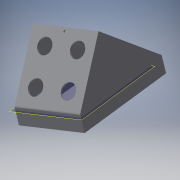
# Autodesk Inventor part: button_angle
Saved by Autodesk Inventor 2016 (Build 200138000, 138)
## iProperties
Created: 2014-10-12
Part Number: button_angle
Material: Generic
Document SubType Name: Modeling
Designer: Alec
Density: 1 g/cm^3
Appearance: Default
Author: Alec
Autodesk Inventor part; units mm, degrees
ref_plane "YZ Plane" through (0, 0, 0) normal (1, 0, 0) x (0, 1, 0)
ref_plane "XZ Plane" through (0, 0, 0) normal (0, 1, 0) x (-1, 0, 0)
ref_plane "XY Plane" through (0, 0, 0) normal (0, 0, 1) x (1, 0, 0)
sketch "Sketch1" plane through (0, 0, 0) normal (0, 1, 0) x (-1, 0, 0)
  line L0 (0, 0) -> (-127, 0)
  line L1 (-127, 0) -> (-127, -6.35)
  line L2 (-127, -6.35) -> (0, -6.35)
  line L3 (0, -6.35) -> (0, 0)
  line L4 (0, -6.35) -> (-6.35, -6.35)
  line L5 (-6.35, -6.35) -> (-6.35, -127)
  line L6 (-6.35, -127) -> (0, -127)
  line L7 (0, -127) -> (0, -6.35)
  line L8 (-127, -6.35) -> (-120.65, -6.35)
  line L9 (-120.65, -6.35) -> (-120.65, -127)
  line L10 (-120.65, -127) -> (-127, -127)
  line L11 (-127, -127) -> (-127, -6.35)
  dimension "d0" = 127
  dimension "d1" = 6.35
  dimension "d2" = 6.35
  dimension "d3" = 120.65
  dimension "d4" = 120.65
  dimension "d5" = 6.35
  constraints: 24 end point, 6 parallel, 3 horizontal, 3 perpendicular
  measures "d0" distance of L1.end L2.end
  measures "d1" distance of L0.end L1.end
  measures "d2" distance of L5.end L6.end
  measures "d3" distance between parallel lines of L2 L6
  measures "d4" distance between parallel lines of L2 L10
  measures "d5" distance between parallel lines of L11 L9
extrude "Extrusion1" add sketch "Sketch1" along normal blind 6.35
sketch "Sketch2" plane through (127, 0, 0) normal (1, 0, 0) x (0, 0, -1)
  line L0 (127, 6.35) -> (120.65, 0)
  line L1 (6.35, 0) -> (127, 0) projected
  line L2 (127, 0) -> (127, 6.35) projected
  line L3 (120.65, 0) -> (127, 0)
  line L4 (127, 0) -> (127, 6.35) projected
  line L5 (127, 6.35) -> (127, 0)
  point P0 (0, 0)
  dimension "d8" = 135
  constraints: 6 end point, 1 collinear, 1 perpendicular, 1 point on line
  measures "d8" angle of L2 L0
extrude "Extrusion2" cut sketch "Sketch2" against normal blind 152.4
sketch "Sketch4" plane through (0, 6.35, 0) normal (0, 1, 0) x (1, 0, 0)
  line L0 (127, 120.65) -> (127, 127)
  line L1 (127, 120.65) -> (127, 127) projected
  line L2 (127, 127) -> (120.65, 127)
  line L3 (120.65, 127) -> (120.65, 120.65)
  line L4 (120.65, 120.65) -> (127, 120.65)
  point P0 (0, 0)
  constraints: 8 end point, 3 perpendicular, 1 collinear
extrude "Extrusion3" cut sketch "Sketch4" against normal blind 152.4
sketch "Sketch5" plane through (0, 6.35, 0) normal (0, 1, 0) x (1, 0, 0)
  line L0 (120.65, 120.65) -> (120.65, 127.0036)
  line L1 (120.65, 127.0036) -> (127.0123, 127.0036)
  line L2 (127.0123, 127.0036) -> (127.0123, 120.65)
  line L3 (127.0123, 120.65) -> (120.65, 120.65)
  point P0 (0, 0)
  constraints: 8 end point, 3 perpendicular, 1 vertical
extrude "Extrusion4" add sketch "Sketch5" against normal blind 152.4
sketch "Sketch6" plane through (0, 6.35, 0) normal (0, 1, 0) x (1, 0, 0)
  line L0 (0, 127) -> (0, 120.65)
  line L1 (0, 127) -> (0, 120.65) projected
  line L2 (0, 120.65) -> (6.35, 120.65)
  line L3 (0, 120.65) -> (6.35, 120.65) projected
  line L4 (6.35, 120.65) -> (6.35, 127)
  line L5 (6.35, 127) -> (0, 127)
  point P0 (0, 0)
  constraints: 8 end point, 2 collinear, 2 perpendicular
extrude "Extrusion5" cut sketch "Sketch6" against normal blind 101.6
sketch "Sketch7" plane through (0, 6.35, 0) normal (0, 1, 0) x (1, 0, 0)
  line L0 (0, 120.65) -> (6.35, 120.65)
  line L1 (6.35, 120.65) -> (6.35, 126.9915)
  line L2 (6.35, 126.9915) -> (0, 126.9915)
  line L3 (0, 126.9915) -> (0, 120.65)
  point P0 (0, 0)
  constraints: 8 end point, 2 parallel, 1 horizontal, 1 perpendicular
extrude "Extrusion6" add sketch "Sketch7" against normal blind 152.4
sketch "Sketch8" plane through (6.35, 0, -6.35) normal (1, 0, 0) x (0, 0, -1)
  line L0 (120.6415, 6.35) -> (120.6415, -146.05) projected
  line L1 (114.3, -146.05) -> (120.6415, -146.05)
  line L2 (120.6415, -146.05) -> (120.6415, -139.7)
  line L3 (120.6415, -139.7) -> (114.3, -139.7)
  line L4 (114.3, -139.7) -> (114.3, -146.05)
  point P0 (-6.35, 0)
  dimension "d19" = 6.35
  constraints: 8 end point, 2 parallel, 1 horizontal, 1 perpendicular, 1 point on line
  measures "d19" distance between parallel lines of L1 L3
extrude "Extrusion7" add sketch "Sketch8" along normal blind 120.65
sketch "Sketch9" plane through (0, 6.35, 0) normal (0, 1, 0) x (1, 0, 0)
  line L0 (0, 126.9915) -> (127, 126.9915)
  line L1 (127, 126.9915) -> (127, 0)
  line L2 (127, 0) -> (0, 0)
  line L3 (0, 0) -> (0, 126.9915)
  constraints: 8 end point, 2 parallel, 1 horizontal, 1 perpendicular
extrude "Extrusion8" add sketch "Sketch9" along normal blind 3.175
sketch "Sketch10" plane through (0, 9.525, 0) normal (0, 1, 0) x (1, 0, 0)
  circle A0 centre (31.75, 95.2415) radius 14.351
  circle A1 centre (95.25, 95.2415) radius 14.351
  circle A2 centre (31.75, 31.75) radius 14.351
  circle A3 centre (95.25, 31.75) radius 14.351
  line L0 (0, 126.9915) -> (0, 0) projected
  line L1 (127, 0) -> (127, 126.9915) projected
  line L2 (127, 126.9915) -> (0, 126.9915) projected
  line L3 (0, 0) -> (127, 0) projected
  dimension "d24" = 28.702
  dimension "d25" = 28.702
  dimension "d26" = 28.702
  dimension "d27" = 28.702
  dimension "d28" = 31.75
  dimension "d29" = 31.75
  dimension "d30" = 31.75
  dimension "d31" = 31.75
  dimension "d32" = 31.75
  dimension "d33" = 31.75
  dimension "d34" = 31.75
  dimension "d35" = 31.75
  constraints: 4 centre point
  measures "d24" diameter of A0
  measures "d25" diameter of A1
  measures "d26" diameter of A2
  measures "d27" diameter of A3
  measures "d28" distance from line of L0 A0.centre
  measures "d29" distance from line of L1 A1.centre
  measures "d30" distance from line of L2 A1.centre
  measures "d31" distance from line of L3 A3.centre
  measures "d32" distance from line of L1 A3.centre
  measures "d33" distance from line of L0 A2.centre
  measures "d34" distance from line of L3 A2.centre
  measures "d35" distance from line of L2 A0.centre
extrude "Extrusion9" cut sketch "Sketch10" against normal blind 25.4 contours A0 | A1 | A2 | A3
ref_plane "Work Plane1" through (0, 0, 0) normal (0, -0.6368859, 0.7709581) x (1, 0, 0)
sketch "Sketch12" plane through (127, 0, -120.65) normal (1, 0, 0) x (0, 0, -1)
  line L0 (6.3415, 9.525) -> (6.3536, -146.05)
  line L1 (6.3536, -146.05) -> (0, -146.05)
  line L2 (6.3536, -146.05) -> (0, -146.05) projected
  line L3 (0, -146.05) -> (-120.65, 0)
  line L4 (-120.65, 0) -> (-120.65, 9.525)
  line L5 (-120.65, 0) -> (-120.65, 9.525) projected
  line L6 (-120.65, 9.525) -> (6.3415, 9.525)
  line L7 (-120.65, 9.525) -> (6.3415, 9.525) projected
  constraints: 10 end point, 3 collinear
extrude "Extrusion11" add sketch "Sketch12" against normal blind 3.175
sketch "Sketch13" plane through (0, -146.05, -126.9915) normal (-1, 0, 0) x (0, 0, 1)
  line L0 (-0.0121, 0) -> (0, 155.575)
  line L1 (0, 155.575) -> (126.9915, 155.575)
  line L2 (126.9915, 155.575) -> (0, 155.575) projected
  line L3 (126.9915, 155.575) -> (126.9915, 146.05)
  line L4 (126.9915, 146.05) -> (6.3415, 0)
  line L5 (6.3415, 0) -> (126.9915, 146.05) projected
  line L6 (6.3415, 0) -> (-0.0121, 0)
  constraints: 10 end point, 2 collinear, 2 perpendicular
extrude "Extrusion12" add sketch "Sketch13" against normal blind 3.175
sketch "Sketch15" plane through (0, 0, 0) normal (0, -0.6368859, 0.7709581) x (1, 0, 0)
  line L0 (127.0123, -189.4387) -> (0, -189.4387)
  line L1 (0, -189.4387) -> (0, 0)
  line L2 (0, 0) -> (127.0123, 0)
  line L3 (127.0123, 0) -> (127.0123, -189.4387)
  constraints: 8 end point, 2 parallel, 1 horizontal, 1 perpendicular
extrude "Extrusion14" add sketch "Sketch15" along normal blind 25.4
sketch "Sketch16" plane through (0, 0, 0) normal (0, 0.6368859, -0.7709581) x (-1, 0, 0)
  line L0 (-6.35, 0.8514) -> (-120.65, 0.8514)
  line L1 (-120.65, 0.8514) -> (-120.65, -186.5598)
  line L2 (-120.65, -186.5598) -> (-6.35, -186.5598)
  line L3 (-6.35, -186.5598) -> (-6.35, 0.8514)
  point P0 (0, 0)
  constraints: 8 end point, 2 parallel, 1 horizontal, 1 perpendicular
extrude "Extrusion15" cut sketch "Sketch16" against normal blind 22.225
sketch "Sketch17" plane through (0, -16.1769, 19.5823) normal (0, 0.7709581, 0.6368859) x (1, 0, 0)
  line L0 (127, 122.4603) -> (127, 25.4) projected
  line L1 (0, 0) -> (127, 0)
  line L2 (127, 0) -> (127, 31.3747)
  line L3 (127, 31.3747) -> (0, 31.3747)
  line L4 (0, 31.3747) -> (0, 0)
  point P0 (0, 25.4)
  constraints: 8 end point, 2 parallel, 1 horizontal, 1 perpendicular, 1 point on line
extrude "Extrusion16" add sketch "Sketch17" along normal blind 7.9375
fillet "Fillet1" radius 3.175 2 edges at (63.5, 9.525, 0) (63.5, 9.9247, 0.4491)
sketch "Sketch19" plane through (0, -146.05, -120.65) normal (0, -0.7709581, -0.6368859) x (1, 0, 0)
  line L0 (127, 25.3989) -> (0, 25.3989)
  line L1 (0, 25.3989) -> (0, -5.2114)
  line L2 (0, -5.2114) -> (127, -5.2114)
  line L3 (127, -5.2114) -> (127, 25.3989)
  point P0 (0, -0.0011)
  constraints: 8 end point, 2 parallel, 1 horizontal, 1 perpendicular
extrude "Extrusion17" add sketch "Sketch19" along normal blind 3.9688
sketch "Sketch23" plane through (0, 9.525, 0) normal (0, 1, 0) x (1, 0, 0)
  line L0 (6.35, 118.8173) -> (120.65, 118.8173) projected
  line L1 (123.825, 126.9915) -> (3.175, 126.9915) projected
  circle A0 centre (63.5, 120.6415) radius 2.54
  line L2 (0, 126.9915) -> (0, 0.9451) projected
  line L3 (127, 0.9451) -> (127, 126.9915) projected
  point P0 (0, 0)
  dimension "d78" = 6.35
  dimension "d80" = 63.5
  dimension "d82" = 5.08
  constraints: 1 centre point
  measures "d78" distance from line of L1 A0.centre
  measures "d80" distance from line of L3 A0.centre
  measures "d82" diameter of A0
extrude "Extrusion21" cut sketch "Sketch23" against normal blind 7.62
body "Solid1"
